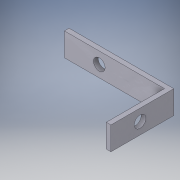
# Autodesk Inventor part: slider_link
Saved by Autodesk Inventor 2019 (Build 230136000, 136)
## iProperties
Created: 2020-02-29
Part Number: slider_link
Material: Stainless Steel AISI 440C, Welded
Document SubType Name: Modeling
Designer: KiranM
Density: 7.8 g/cm^3
Appearance: Weld - Stainless Steel
Author: KiranM
Autodesk Inventor part; units mm, degrees
ref_plane "YZ Plane" through (0, 0, 0) normal (1, 0, 0) x (0, 1, 0)
ref_plane "XZ Plane" through (0, 0, 0) normal (0, 1, 0) x (-1, 0, 0)
ref_plane "XY Plane" through (0, 0, 0) normal (0, 0, 1) x (1, 0, 0)
sketch "Sketch1" plane through (0, 0, 0) normal (0, 0, 1) x (1, 0, 0)
  line L0 (0, 0) -> (45, 0)
  line L1 (45, 0) -> (45, -10)
  line L2 (45, -10) -> (0, -10)
  line L3 (0, -10) -> (0, 0)
  line L4 (45, 0) -> (48.2934, 0)
  line L5 (48.2934, 0) -> (48.2934, -10)
  line L6 (48.2934, -10) -> (45, -10)
  line L7 (45, -10) -> (45, 0)
  constraints: 16 end point, 4 parallel, 2 horizontal, 2 perpendicular, 1 point on line
extrude "Extrusion1" add sketch "Sketch1" along normal blind 2 contours L0 L1 L2 L3
sketch "Sketch2" plane through (0, 0, 2) normal (0, 0, 1) x (1, 0, 0)
  line L0 (0, 0) -> (0, -5)
  circle A0 centre (15, -5) radius 2.5
  constraints: 2 end point, 1 centre point, 1 vertical
extrude "Extrusion2" cut sketch "Sketch2" against normal blind 2
sketch "Sketch3" plane through (0, 0, 2) normal (0, 0, 1) x (1, 0, 0)
  line L0 (45, -10) -> (45, 0) projected
  line L1 (45, 0) -> (43, 0)
  line L2 (45, 0) -> (0, 0) projected
  line L3 (43, 0) -> (43, -10)
  line L4 (0, -10) -> (45, -10) projected
  line L5 (43, -10) -> (45, -10)
  line L6 (45, -10) -> (45, 0)
  dimension "d10" = 2
  constraints: 8 end point, 2 perpendicular, 1 collinear, 1 point on line
  measures "d10" distance between parallel lines of L3 L0
extrude "Extrusion3" add sketch "Sketch3" along normal blind 25
sketch "Sketch4" plane through (43, -10, 2) normal (-1, 0, 0) x (0, 0, 1)
  line L0 (25, 0) -> (25, 10) projected
  circle A0 centre (12.5, 5) radius 2.5
  point P0 (-2, 10)
  constraints: 1 centre point
extrude "Extrusion4" cut sketch "Sketch4" against normal blind 25
body "Solid1"
